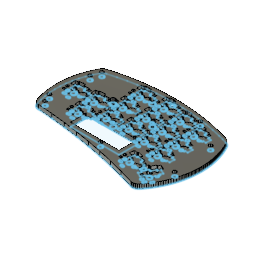
wubmeat-back (Autodesk Fusion 360 design; units mm, degrees)
Autodesk Fusion 360 part; units mm, degrees
(part 1 of 7)
sketch "test (1)" plane through (0, 0, 0) normal (0, 0, 1) x (1, 0, 0)
  line L0 (83.4424, 85.5345) -> (83.3623, 80.9353)
  line L1 (97.0028, 84.2973) -> (92.5034, 84.3759)
  line L2 (96.886, 77.5985) -> (96.9026, 78.5483)
  spline S0 degree 3 poles (84.2605, 76.4435) (84.4967, 76.6798) (84.6294, 77.0003) (84.6294, 77.3344) knots 0 0 0 0 1 1 1 1
  spline S1 degree 3 poles (83.369, 76.0746) (83.7034, 76.0744) (84.024, 76.2072) (84.2605, 76.4435) knots 0 0 0 0 1 1 1 1
  spline S2 degree 3 poles (84.6294, 77.3344) (84.6294, 77.6686) (84.4967, 77.989) (84.2605, 78.2253) knots 0 0 0 0 1 1 1 1
  line L3 (99.1805, 61.506) -> (99.2606, 66.1052)
  spline S3 degree 3 poles (83.369, 78.5943) (83.7034, 78.5945) (84.024, 78.4617) (84.2605, 78.2253) knots 0 0 0 0 1 1 1 1
  line L4 (92.03, 85.8843) -> (91.5386, 86.3933)
  line L5 (91.5386, 86.3933) -> (86.5394, 86.4806)
  spline S4 degree 3 poles (84.2605, 78.2253) (84.4967, 77.989) (84.6294, 77.6686) (84.6294, 77.3344) knots 0 0 0 0 1 1 1 1
  line L6 (90.0901, 60.7148) -> (96.5894, 60.6011)
  spline S5 degree 3 poles (84.2605, 76.4435) (84.024, 76.2072) (83.7034, 76.0744) (83.369, 76.0746) knots 0 0 0 0 1 1 1 1
  spline S6 degree 3 poles (83.369, 76.0746) (83.0349, 76.0746) (82.7144, 76.2073) (82.4781, 76.4435) knots 0 0 0 0 1 1 1 1
  line L7 (86.002, 85.4895) -> (83.4424, 85.5345)
  spline S7 degree 3 poles (89.6162, 62.5901) (89.8898, 62.3539) (90.0648, 62.0236) (90.1066, 61.6646) knots 0 0 0 0 1 1 1 1
  line L8 (83.3623, 80.9353) -> (86.3916, 80.882)
  line L9 (90.4038, 78.662) -> (90.3867, 77.7122)
  spline S8 degree 3 poles (82.4781, 76.4435) (82.7144, 76.2073) (83.0349, 76.0746) (83.369, 76.0746) knots 0 0 0 0 1 1 1 1
  spline S9 degree 3 poles (84.6294, 77.3344) (84.6294, 77.0003) (84.4967, 76.6798) (84.2605, 76.4435) knots 0 0 0 0 1 1 1 1
  line L10 (83.369, 78.5943) -> (83.369, 78.5943)
  spline S10 degree 3 poles (91.8543, 67.5299) (91.762, 67.6256) (91.712, 67.7545) (91.7158, 67.8875) knots 0 0 0 0 1 1 1 1
  line L11 (96.6861, 66.1501) -> (96.7062, 67.2999)
  spline S11 degree 3 poles (89.8984, 79.0222) (89.7425, 79.1123) (89.5756, 79.1816) (89.4017, 79.2284) knots 0 0 0 0 1 1 1 1
  line L12 (91.2419, 69.3959) -> (86.2428, 69.4832)
  spline S12 degree 3 poles (88.9258, 79.9379) (89.2871, 79.9488) (89.6393, 79.8238) (89.9128, 79.5875) knots 0 0 0 0 1 1 1 1
  line L13 (96.606, 61.5509) -> (99.1805, 61.506)
  line L14 (91.7334, 68.8869) -> (91.2419, 69.3959)
  line L15 (86.0102, 85.9696) -> (86.002, 85.4895)
  spline S13 degree 3 poles (89.9128, 79.5875) (90.1866, 79.3514) (90.3618, 79.0211) (90.4038, 78.662) knots 0 0 0 0 1 1 1 1
  line L16 (99.2606, 66.1052) -> (96.6861, 66.1501)
  line L17 (99.4771, 78.5034) -> (99.5572, 83.1026)
  spline S14 degree 3 poles (83.369, 78.5943) (83.0349, 78.5943) (82.7144, 78.4616) (82.4781, 78.2253) knots 0 0 0 0 1 1 1 1
  spline S15 degree 3 poles (92.1509, 84.5273) (92.0586, 84.623) (92.0087, 84.7519) (92.0124, 84.8849) knots 0 0 0 0 1 1 1 1
  line L18 (86.5394, 86.4807) -> (86.0102, 85.9696)
  spline S16 degree 3 poles (82.4781, 78.2253) (82.2419, 77.989) (82.1092, 77.6686) (82.1092, 77.3344) knots 0 0 0 0 1 1 1 1
  line L19 (83.369, 78.5943) -> (83.369, 78.5943)
  spline S17 degree 3 poles (82.1092, 77.3344) (82.1092, 77.6686) (82.2419, 77.989) (82.4781, 78.2253) knots 0 0 0 0 1 1 1 1
  spline S18 degree 3 poles (82.4781, 78.2253) (82.7144, 78.4616) (83.0349, 78.5943) (83.369, 78.5943) knots 0 0 0 0 1 1 1 1
  line L20 (96.9827, 83.1475) -> (97.0028, 84.2973)
  spline S19 degree 3 poles (90.4027, 78.5943) (90.3779, 78.6287) (90.3521, 78.6623) (90.3252, 78.6951) knots 0 0 0 0 1 1 1 1
  spline S20 degree 3 poles (84.2605, 78.2253) (84.024, 78.4617) (83.7034, 78.5945) (83.369, 78.5943) knots 0 0 0 0 1 1 1 1
  spline S21 degree 3 poles (90.3252, 78.6951) (90.1978, 78.8223) (90.0543, 78.9323) (89.8984, 79.0222) knots 0 0 0 0 1 1 1 1
  line L21 (90.1066, 61.6646) -> (90.0901, 60.7148)
  spline S22 degree 3 poles (87.4117, 78.6951) (87.0254, 78.3087) (86.8085, 77.7847) (86.8086, 77.2383) knots 0 0 0 0 1 1 1 1
  line L22 (99.5572, 83.1026) -> (96.9827, 83.1475)
  spline S23 degree 3 poles (88.8684, 79.2987) (88.322, 79.2986) (87.798, 79.0815) (87.4117, 78.6951) knots 0 0 0 0 1 1 1 1
  spline S24 degree 3 poles (89.4017, 79.2284) (89.2278, 79.275) (89.0485, 79.2986) (88.8684, 79.2987) knots 0 0 0 0 1 1 1 1
  spline S25 degree 3 poles (86.8086, 77.2383) (86.8085, 76.692) (87.0254, 76.168) (87.4117, 75.7816) knots 0 0 0 0 1 1 1 1
  spline S26 degree 3 poles (82.4781, 76.4435) (82.2419, 76.6798) (82.1092, 77.0003) (82.1092, 77.3344) knots 0 0 0 0 1 1 1 1
  spline S27 degree 3 poles (92.5034, 84.3759) (92.3703, 84.3769) (92.2433, 84.4315) (92.1509, 84.5273) knots 0 0 0 0 1 1 1 1
  spline S28 degree 3 poles (92.2067, 67.3785) (92.0737, 67.3795) (91.9467, 67.4341) (91.8543, 67.5299) knots 0 0 0 0 1 1 1 1
  spline S29 degree 3 poles (87.4117, 75.7816) (87.7981, 75.3953) (88.3221, 75.1784) (88.8684, 75.1785) knots 0 0 0 0 1 1 1 1
  line L23 (96.9026, 78.5483) -> (99.4771, 78.5034)
  line L24 (92.0124, 84.8849) -> (92.03, 85.8843)
  spline S30 degree 3 poles (82.1092, 77.3344) (82.1092, 77.0003) (82.2419, 76.6798) (82.4781, 76.4435) knots 0 0 0 0 1 1 1 1
  line L25 (90.3867, 77.7122) -> (96.886, 77.5985)
  line L26 (96.5894, 60.6011) -> (96.606, 61.5509)
  line L27 (87.3259, 79.9658) -> (88.9258, 79.9379)
  line L28 (86.3916, 80.882) -> (87.3259, 79.9658)
  line L29 (91.7158, 67.8875) -> (91.7334, 68.8869)
  spline S31 degree 3 poles (90.3252, 75.7816) (90.4524, 75.9089) (90.5624, 76.0524) (90.6523, 76.2084) knots 0 0 0 0 1 1 1 1
  line L30 (33.6537, 35.5701) -> (33.5768, 36.4532)
  spline S32 degree 3 poles (27.1038, 35.6595) (26.9779, 35.7005) (26.8465, 35.7214) (26.7141, 35.7215) knots 0 0 0 0 1 1 1 1
  line L31 (90.8673, 77.7039) -> (90.3867, 77.7122)
  spline S33 degree 3 poles (70.73, 73.4437) (71.0515, 73.4438) (71.3486, 73.6154) (71.5093, 73.8938) knots 0 0 0 0 1 1 1 1
  spline S34 degree 3 poles (87.3254, 70.9152) (87.1701, 71.1959) (87.176, 71.5381) (87.3409, 71.8133) knots 0 0 0 0 1 1 1 1
  line L32 (89.4048, 70.4279) -> (88.0949, 70.4511)
  spline S35 degree 3 poles (34.1829, 34.4074) (34.2296, 34.5813) (34.2532, 34.7606) (34.2532, 34.9407) knots 0 0 0 0 1 1 1 1
  spline S36 degree 3 poles (34.1829, 35.474) (34.1656, 35.5204) (34.1467, 35.5663) (34.1261, 35.6114) knots 0 0 0 0 1 1 1 1
  spline S37 degree 3 poles (90.1898, 70.8651) (90.0248, 70.5898) (89.7257, 70.4232) (89.4048, 70.4279) knots 0 0 0 0 1 1 1 1
  line L33 (72.5852, 72.4438) -> (73.0849, 71.9436)
  spline S38 degree 3 poles (27.9125, 34.8507) (27.8717, 34.9764) (27.8113, 35.0948) (27.7337, 35.2016) knots 0 0 0 0 1 1 1 1
  spline S39 degree 3 poles (88.8684, 75.1785) (89.0485, 75.1785) (89.2278, 75.2021) (89.4017, 75.2488) knots 0 0 0 0 1 1 1 1
  spline S40 degree 3 poles (27.7337, 33.7206) (27.8114, 33.8276) (27.8717, 33.9462) (27.9125, 34.072) knots 0 0 0 0 1 1 1 1
  spline S41 degree 3 poles (27.974, 34.4611) (27.9741, 34.5934) (27.9533, 34.7249) (27.9125, 34.8507) knots 0 0 0 0 1 1 1 1
  line L34 (69.42, 73.4437) -> (70.73, 73.4437)
  spline S42 degree 3 poles (68.6407, 73.8938) (68.8015, 73.6154) (69.0985, 73.4438) (69.42, 73.4437) knots 0 0 0 0 1 1 1 1
  spline S43 degree 3 poles (33.9772, 33.9107) (34.0672, 34.0666) (34.1363, 34.2335) (34.1829, 34.4074) knots 0 0 0 0 1 1 1 1
  line L35 (34.1261, 35.6114) -> (33.6537, 35.5701)
  spline S44 degree 3 poles (68.6407, 74.7935) (68.4801, 74.5151) (68.4801, 74.1722) (68.6407, 73.8938) knots 0 0 0 0 1 1 1 1
  spline S45 degree 3 poles (87.3409, 71.8133) (87.506, 72.0887) (87.8053, 72.2553) (88.1264, 72.2505) knots 0 0 0 0 1 1 1 1
  spline S46 degree 3 poles (93.3219, 77.661) (93.2123, 77.5064) (93.139, 77.3291) (93.1075, 77.1422) knots 0 0 0 0 1 1 1 1
  line L36 (67.585, 72.4438) -> (72.5852, 72.4438)
  spline S47 degree 3 poles (26.7141, 35.7215) (26.3799, 35.7214) (26.0594, 35.5884) (25.8232, 35.352) knots 0 0 0 0 1 1 1 1
  line L37 (26.7141, 35.7215) -> (26.7141, 35.7215)
  line L38 (73.0849, 71.9436) -> (73.0849, 70.9436)
  spline S48 degree 3 poles (89.4017, 75.2488) (89.5756, 75.2954) (89.7425, 75.3645) (89.8984, 75.4545) knots 0 0 0 0 1 1 1 1
  spline S49 degree 3 poles (90.8585, 76.705) (90.905, 76.879) (90.9284, 77.0583) (90.9283, 77.2383) knots 0 0 0 0 1 1 1 1
  spline S50 degree 3 poles (25.8232, 33.5702) (26.0595, 33.3339) (26.38, 33.2012) (26.7141, 33.2012) knots 0 0 0 0 1 1 1 1
  spline S51 degree 3 poles (33.2233, 33.1568) (33.3791, 33.2467) (33.5224, 33.3567) (33.6496, 33.4839) knots 0 0 0 0 1 1 1 1
  spline S52 degree 3 poles (88.0949, 70.4511) (87.774, 70.4576) (87.4808, 70.6344) (87.3254, 70.9152) knots 0 0 0 0 1 1 1 1
  spline S53 degree 3 poles (25.4543, 34.4611) (25.4542, 34.127) (25.587, 33.8065) (25.8232, 33.5702) knots 0 0 0 0 1 1 1 1
  spline S54 degree 3 poles (89.8984, 75.4545) (90.0543, 75.5444) (90.1978, 75.6543) (90.3252, 75.7816) knots 0 0 0 0 1 1 1 1
  spline S55 degree 3 poles (26.7141, 33.2012) (26.8464, 33.2011) (26.9779, 33.2219) (27.1038, 33.2627) knots 0 0 0 0 1 1 1 1
  spline S56 degree 3 poles (27.9125, 34.072) (27.9533, 34.1977) (27.974, 34.329) (27.974, 34.4611) knots 0 0 0 0 1 1 1 1
  spline S57 degree 3 poles (27.4546, 35.4807) (27.3478, 35.5583) (27.2294, 35.6186) (27.1038, 35.6595) knots 0 0 0 0 1 1 1 1
  spline S58 degree 3 poles (93.4764, 76.2513) (93.7129, 76.0149) (94.0335, 75.8822) (94.3679, 75.8823) knots 0 0 0 0 1 1 1 1
  spline S59 degree 3 poles (90.9283, 77.2383) (90.9258, 77.3953) (90.9053, 77.5516) (90.8673, 77.7039) knots 0 0 0 0 1 1 1 1
  spline S60 degree 3 poles (34.2532, 34.9407) (34.2532, 35.1207) (34.2296, 35.3) (34.1829, 35.474) knots 0 0 0 0 1 1 1 1
  spline S61 degree 3 poles (25.8232, 35.352) (25.587, 35.1157) (25.4542, 34.7952) (25.4543, 34.4611) knots 0 0 0 0 1 1 1 1
  spline S62 degree 3 poles (33.6496, 33.4839) (33.777, 33.6112) (33.8872, 33.7548) (33.9772, 33.9107) knots 0 0 0 0 1 1 1 1
  spline S63 degree 3 poles (69.42, 75.2436) (69.0985, 75.2435) (68.8015, 75.072) (68.6407, 74.7935) knots 0 0 0 0 1 1 1 1
  spline S64 degree 3 poles (93.1075, 77.1422) (93.1075, 76.8081) (93.2402, 76.4876) (93.4764, 76.2513) knots 0 0 0 0 1 1 1 1
  spline S65 degree 3 poles (90.6523, 76.2084) (90.7425, 76.3642) (90.8118, 76.5312) (90.8585, 76.705) knots 0 0 0 0 1 1 1 1
  spline S66 degree 3 poles (27.1038, 33.2627) (27.2294, 33.3037) (27.3478, 33.3642) (27.4546, 33.442) knots 0 0 0 0 1 1 1 1
  spline S67 degree 3 poles (90.2058, 71.7637) (90.3612, 71.4828) (90.3551, 71.1403) (90.1898, 70.8651) knots 0 0 0 0 1 1 1 1
  line L39 (90.3867, 77.7122) -> (90.4027, 78.5943)
  spline S68 degree 3 poles (89.4359, 72.2278) (89.7569, 72.2215) (90.0503, 72.0447) (90.2058, 71.7637) knots 0 0 0 0 1 1 1 1
  spline S69 degree 3 poles (27.7337, 35.2016) (27.6559, 35.3087) (27.5617, 35.4029) (27.4546, 35.4807) knots 0 0 0 0 1 1 1 1
  spline S70 degree 3 poles (27.4546, 33.442) (27.5617, 33.5197) (27.6559, 33.6137) (27.7337, 33.7206) knots 0 0 0 0 1 1 1 1
  line L40 (78.0851, 70.4434) -> (78.0851, 69.2936)
  line L41 (64.5051, 66.8436) -> (64.5051, 71.4438)
  line L42 (49.491, 73.2034) -> (49.491, 73.2034)
  spline S71 degree 3 poles (49.491, 73.2034) (49.8122, 73.2203) (50.1179, 73.0644) (50.293, 72.7947) knots 0 0 0 0 1 1 1 1
  spline S72 degree 3 poles (50.3401, 71.896) (50.1941, 71.6094) (49.9063, 71.4224) (49.5851, 71.4056) knots 0 0 0 0 1 1 1 1
  line L43 (49.5851, 71.4056) -> (48.2771, 71.3374)
  spline S73 degree 3 poles (102.8154, 73.1207) (102.9225, 73.0431) (103.0166, 72.9491) (103.0944, 72.8422) knots 0 0 0 0 1 1 1 1
  spline S74 degree 3 poles (103.2733, 72.4908) (103.314, 72.3651) (103.3348, 72.2338) (103.3347, 72.1017) knots 0 0 0 0 1 1 1 1
  spline S75 degree 3 poles (102.9658, 71.2103) (102.7295, 70.974) (102.409, 70.8413) (102.0749, 70.8413) knots 0 0 0 0 1 1 1 1
  spline S76 degree 3 poles (50.293, 72.7947) (50.4681, 72.525) (50.486, 72.1825) (50.3401, 71.896) knots 0 0 0 0 1 1 1 1
  line L44 (67.0651, 71.4438) -> (67.0651, 71.9234)
  spline S77 degree 3 poles (49.5851, 71.4056) (49.9063, 71.4224) (50.1941, 71.6094) (50.3401, 71.896) knots 0 0 0 0 1 1 1 1
  spline S78 degree 3 poles (100.815, 72.1017) (100.815, 72.4358) (100.9477, 72.7563) (101.184, 72.9926) knots 0 0 0 0 1 1 1 1
  line L45 (73.5851, 70.4434) -> (78.0851, 70.4434)
  spline S79 degree 3 poles (71.0783, 65.6106) (70.8006, 65.842) (70.4462, 65.9607) (70.0851, 65.9434) knots 0 0 0 0 1 1 1 1
  line L46 (68.4852, 65.9434) -> (67.5349, 66.8436)
  spline S80 degree 3 poles (48.1826, 73.1347) (47.8615, 73.1177) (47.574, 72.9308) (47.4281, 72.6443) knots 0 0 0 0 1 1 1 1
  line L47 (48.2771, 71.3374) -> (49.5851, 71.4056)
  line L48 (48.1826, 73.1347) -> (49.491, 73.2034)
  spline S81 degree 3 poles (102.4645, 73.2995) (102.5901, 73.2587) (102.7085, 73.1984) (102.8154, 73.1207) knots 0 0 0 0 1 1 1 1
  spline S82 degree 3 poles (103.3347, 72.1017) (103.3349, 71.7674) (103.2022, 71.4467) (102.9658, 71.2103) knots 0 0 0 0 1 1 1 1
  spline S83 degree 3 poles (71.5853, 64.6934) (71.5371, 65.0518) (71.3562, 65.3792) (71.0783, 65.6106) knots 0 0 0 0 1 1 1 1
  line L49 (78.0851, 64.6934) -> (78.0851, 63.7435)
  spline S84 degree 3 poles (101.184, 71.2103) (100.9476, 71.4467) (100.8149, 71.7674) (100.815, 72.1017) knots 0 0 0 0 1 1 1 1
  spline S85 degree 3 poles (73.2301, 70.5886) (73.3241, 70.4944) (73.4521, 70.4421) (73.5851, 70.4434) knots 0 0 0 0 1 1 1 1
  line L50 (49.491, 73.2034) -> (48.1826, 73.1347)
  spline S86 degree 3 poles (102.0749, 73.3616) (102.2072, 73.3615) (102.3387, 73.3405) (102.4645, 73.2995) knots 0 0 0 0 1 1 1 1
  spline S87 degree 3 poles (102.0749, 70.8413) (101.7407, 70.8413) (101.4203, 70.974) (101.184, 71.2103) knots 0 0 0 0 1 1 1 1
  line L51 (78.0851, 63.7435) -> (71.5853, 63.7435)
  line L52 (71.5853, 63.7435) -> (71.5853, 64.6934)
  line L53 (80.6602, 69.2936) -> (80.6602, 64.6934)
  line L54 (64.5051, 71.4438) -> (67.0651, 71.4438)
  line L55 (67.0651, 71.9234) -> (67.585, 72.4438)
  line L56 (67.5349, 66.8436) -> (64.5051, 66.8436)
  spline S88 degree 3 poles (47.4751, 71.7456) (47.6504, 71.4761) (47.9561, 71.3204) (48.2771, 71.3374) knots 0 0 0 0 1 1 1 1
  spline S89 degree 3 poles (47.4751, 71.7456) (47.3001, 72.0153) (47.2821, 72.3578) (47.4281, 72.6443) knots 0 0 0 0 1 1 1 1
  spline S90 degree 3 poles (103.0944, 72.8422) (103.1721, 72.7352) (103.2325, 72.6166) (103.2733, 72.4908) knots 0 0 0 0 1 1 1 1
  spline S91 degree 3 poles (50.3401, 71.896) (50.486, 72.1825) (50.4681, 72.525) (50.293, 72.7947) knots 0 0 0 0 1 1 1 1
  line L57 (80.6602, 64.6934) -> (78.0851, 64.6934)
  line L58 (70.0851, 65.9434) -> (68.4852, 65.9434)
  line L59 (88.1264, 72.2505) -> (88.1264, 72.2505)
  spline S92 degree 3 poles (73.0849, 70.9436) (73.0836, 70.8106) (73.136, 70.6826) (73.2301, 70.5886) knots 0 0 0 0 1 1 1 1
  line L60 (78.0851, 69.2936) -> (80.6602, 69.2936)
  spline S93 degree 3 poles (48.2771, 71.3374) (47.9561, 71.3204) (47.6504, 71.4761) (47.4751, 71.7456) knots 0 0 0 0 1 1 1 1
  spline S94 degree 3 poles (47.4281, 72.6443) (47.574, 72.9308) (47.8615, 73.1177) (48.1826, 73.1347) knots 0 0 0 0 1 1 1 1
  spline S95 degree 3 poles (50.293, 72.7947) (50.1179, 73.0644) (49.8122, 73.2203) (49.491, 73.2034) knots 0 0 0 0 1 1 1 1
  spline S96 degree 3 poles (47.4281, 72.6443) (47.2821, 72.3578) (47.3001, 72.0153) (47.4751, 71.7456) knots 0 0 0 0 1 1 1 1
  spline S97 degree 3 poles (110.1416, 22.527) (109.6775, 22.5269) (109.2325, 22.3425) (108.9044, 22.0143) knots 0 0 0 0 1 1 1 1
  spline S98 degree 3 poles (108.9044, 19.5395) (109.2325, 19.2114) (109.6775, 19.027) (110.1416, 19.0269) knots 0 0 0 0 1 1 1 1
  spline S99 degree 3 poles (108.9044, 22.0143) (108.5762, 21.6861) (108.3918, 21.2409) (108.3918, 20.7767) knots 0 0 0 0 1 1 1 1
  spline S100 degree 3 poles (111.3792, 19.5395) (111.7074, 19.8676) (111.8917, 20.3126) (111.8918, 20.7767) knots 0 0 0 0 1 1 1 1
  line L61 (102.0749, 73.3616) -> (102.0749, 73.3616)
  spline S101 degree 3 poles (111.8918, 20.7767) (111.8918, 20.9297) (111.8716, 21.0821) (111.8319, 21.2299) knots 0 0 0 0 1 1 1 1
  spline S102 degree 3 poles (111.017, 22.2923) (110.8845, 22.3688) (110.7425, 22.4275) (110.5948, 22.467) knots 0 0 0 0 1 1 1 1
  spline S103 degree 3 poles (110.5948, 22.467) (110.447, 22.5067) (110.2946, 22.5269) (110.1416, 22.527) knots 0 0 0 0 1 1 1 1
  spline S104 degree 3 poles (111.6572, 21.6516) (111.5808, 21.7841) (111.4873, 21.9061) (111.3792, 22.0143) knots 0 0 0 0 1 1 1 1
  line L62 (110.1416, 22.527) -> (110.1416, 22.527)
  spline S105 degree 3 poles (102.6366, 18.7768) (102.4002, 18.5406) (102.2672, 18.2201) (102.2671, 17.8859) knots 0 0 0 0 1 1 1 1
  spline S106 degree 3 poles (103.5275, 19.1458) (103.1934, 19.1458) (102.8729, 19.013) (102.6366, 18.7768) knots 0 0 0 0 1 1 1 1
  spline S107 degree 3 poles (102.2671, 17.8859) (102.2672, 17.5517) (102.4002, 17.2312) (102.6366, 16.995) knots 0 0 0 0 1 1 1 1
  spline S108 degree 3 poles (108.3918, 20.7767) (108.3919, 20.3126) (108.5763, 19.8676) (108.9044, 19.5395) knots 0 0 0 0 1 1 1 1
  spline S109 degree 3 poles (111.3792, 22.0143) (111.2711, 22.1224) (111.1493, 22.2159) (111.017, 22.2923) knots 0 0 0 0 1 1 1 1
  spline S110 degree 3 poles (111.8319, 21.2299) (111.7923, 21.3775) (111.7336, 21.5192) (111.6572, 21.6516) knots 0 0 0 0 1 1 1 1
  spline S111 degree 3 poles (103.5275, 16.626) (103.8616, 16.626) (104.1821, 16.7587) (104.4184, 16.995) knots 0 0 0 0 1 1 1 1
  spline S112 degree 3 poles (110.1416, 19.0269) (110.6058, 19.0269) (111.051, 19.2113) (111.3792, 19.5395) knots 0 0 0 0 1 1 1 1
  spline S113 degree 3 poles (102.6366, 16.995) (102.8729, 16.7587) (103.1934, 16.626) (103.5275, 16.626) knots 0 0 0 0 1 1 1 1
  spline S114 degree 3 poles (104.7874, 17.8859) (104.7874, 18.018) (104.7666, 18.1493) (104.7259, 18.275) knots 0 0 0 0 1 1 1 1
  spline S115 degree 3 poles (101.184, 72.9926) (101.4203, 73.2288) (101.7407, 73.3616) (102.0749, 73.3616) knots 0 0 0 0 1 1 1 1
  line L63 (88.1264, 72.2505) -> (89.4359, 72.2278)
  spline S116 degree 3 poles (118.1344, 12.6071) (118.0087, 12.6481) (117.8774, 12.669) (117.7452, 12.6692) knots 0 0 0 0 1 1 1 1
  line L64 (117.7452, 12.6692) -> (117.7452, 12.6692)
  spline S117 degree 3 poles (117.7452, 12.6692) (117.8774, 12.669) (118.0087, 12.6481) (118.1344, 12.6071) knots 0 0 0 0 1 1 1 1
  spline S118 degree 3 poles (103.9166, 19.0843) (103.7909, 19.125) (103.6596, 19.1458) (103.5275, 19.1458) knots 0 0 0 0 1 1 1 1
  spline S119 degree 3 poles (96.6716, 20.3922) (96.2853, 20.0058) (96.0684, 19.4818) (96.0685, 18.9354) knots 0 0 0 0 1 1 1 1
  line L65 (44.388, 75.0385) -> (43.0795, 74.9702)
  spline S120 degree 3 poles (119.0051, 11.4088) (119.0051, 11.0746) (118.8724, 10.7542) (118.6361, 10.5179) knots 0 0 0 0 1 1 1 1
  line L66 (131.3718, 31.3068) -> (131.3718, 31.3068)
  spline S121 degree 3 poles (104.5466, 18.6264) (104.4689, 18.7335) (104.3749, 18.8276) (104.268, 18.9055) knots 0 0 0 0 1 1 1 1
  spline S122 degree 3 poles (42.3721, 73.5812) (42.5472, 73.3114) (42.8529, 73.1556) (43.1741, 73.1724) knots 0 0 0 0 1 1 1 1
  spline S123 degree 3 poles (104.4184, 16.995) (104.6547, 17.2313) (104.7874, 17.5517) (104.7874, 17.8859) knots 0 0 0 0 1 1 1 1
  spline S124 degree 3 poles (116.4848, 11.4088) (116.485, 11.743) (116.6179, 12.0635) (116.8543, 12.2997) knots 0 0 0 0 1 1 1 1
  spline S125 degree 3 poles (132.6089, 30.7941) (132.5008, 30.9022) (132.379, 30.9957) (132.2467, 31.0722) knots 0 0 0 0 1 1 1 1
  spline S126 degree 3 poles (118.4858, 12.4283) (118.5927, 12.3505) (118.6867, 12.2564) (118.7643, 12.1493) knots 0 0 0 0 1 1 1 1
  spline S127 degree 3 poles (116.8543, 10.5179) (116.6179, 10.7541) (116.485, 11.0746) (116.4848, 11.4088) knots 0 0 0 0 1 1 1 1
  spline S128 degree 3 poles (116.8543, 12.2997) (117.0905, 12.5361) (117.411, 12.669) (117.7452, 12.6692) knots 0 0 0 0 1 1 1 1
  spline S129 degree 3 poles (96.0685, 18.9354) (96.0684, 18.3891) (96.2853, 17.8651) (96.6716, 17.4787) knots 0 0 0 0 1 1 1 1
  spline S130 degree 3 poles (44.482, 73.2412) (44.8032, 73.258) (45.0911, 73.4449) (45.237, 73.7316) knots 0 0 0 0 1 1 1 1
  spline S131 degree 3 poles (125.6832, 15.2519) (125.3626, 15.2296) (125.0781, 15.038) (124.937, 14.7491) knots 0 0 0 0 1 1 1 1
  spline S132 degree 3 poles (43.9735, 78.7654) (43.7372, 79.0016) (43.4168, 79.1343) (43.0826, 79.1343) knots 0 0 0 0 1 1 1 1
  line L67 (103.5275, 19.1458) -> (103.5275, 19.1458)
  spline S133 degree 3 poles (43.0795, 74.9702) (42.7585, 74.9533) (42.4709, 74.7663) (42.3251, 74.4798) knots 0 0 0 0 1 1 1 1
  spline S134 degree 3 poles (132.2467, 31.0722) (132.1142, 31.1488) (131.9723, 31.2077) (131.8245, 31.2473) knots 0 0 0 0 1 1 1 1
  line L68 (124.937, 14.7491) -> (124.3629, 13.5719)
  spline S135 degree 3 poles (124.3629, 13.5719) (124.223, 13.283) (124.2476, 12.9413) (124.4275, 12.6754) knots 0 0 0 0 1 1 1 1
  line L69 (117.7452, 12.6692) -> (117.7452, 12.6692)
  spline S136 degree 3 poles (130.1341, 28.3194) (130.4624, 27.9911) (130.9076, 27.8067) (131.3718, 27.8067) knots 0 0 0 0 1 1 1 1
  spline S137 degree 3 poles (124.4275, 12.6754) (124.6072, 12.4096) (124.9147, 12.2596) (125.2347, 12.2816) knots 0 0 0 0 1 1 1 1
  line L70 (125.9809, 12.7828) -> (126.555, 13.96)
  line L71 (44.388, 75.0385) -> (44.388, 75.0385)
  spline S138 degree 3 poles (96.6716, 17.4787) (97.0579, 17.0922) (97.5819, 16.8751) (98.1283, 16.8751) knots 0 0 0 0 1 1 1 1
  spline S139 degree 3 poles (99.1583, 17.1516) (99.3142, 17.2415) (99.4577, 17.3515) (99.5851, 17.4787) knots 0 0 0 0 1 1 1 1
  spline S140 degree 3 poles (42.3251, 74.4798) (42.1791, 74.1934) (42.197, 73.8508) (42.3721, 73.5812) knots 0 0 0 0 1 1 1 1
  line L72 (43.1741, 73.1724) -> (44.482, 73.2412)
  spline S141 degree 3 poles (104.268, 18.9055) (104.161, 18.9831) (104.0424, 19.0435) (103.9166, 19.0843) knots 0 0 0 0 1 1 1 1
  spline S142 degree 3 poles (99.9122, 17.9055) (100.0023, 18.0613) (100.0717, 18.2283) (100.1184, 18.4021) knots 0 0 0 0 1 1 1 1
  spline S143 degree 3 poles (45.237, 73.7316) (45.383, 74.018) (45.365, 74.3606) (45.19, 74.6302) knots 0 0 0 0 1 1 1 1
  spline S144 degree 3 poles (98.1283, 16.8751) (98.3084, 16.8751) (98.4877, 16.8987) (98.6616, 16.9454) knots 0 0 0 0 1 1 1 1
  spline S145 degree 3 poles (43.9735, 76.9836) (44.2098, 77.2199) (44.3425, 77.5403) (44.3425, 77.8745) knots 0 0 0 0 1 1 1 1
  spline S146 degree 3 poles (99.5851, 17.4787) (99.7123, 17.6061) (99.8223, 17.7496) (99.9122, 17.9055) knots 0 0 0 0 1 1 1 1
  spline S147 degree 3 poles (132.6089, 28.3194) (132.9372, 28.6476) (133.1216, 29.0928) (133.1215, 29.557) knots 0 0 0 0 1 1 1 1
  spline S148 degree 3 poles (133.1215, 29.557) (133.1216, 29.7099) (133.1016, 29.862) (133.0621, 30.0097) knots 0 0 0 0 1 1 1 1
  spline S149 degree 3 poles (130.1341, 30.7941) (129.806, 30.466) (129.6216, 30.021) (129.6215, 29.557) knots 0 0 0 0 1 1 1 1
  spline S150 degree 3 poles (133.0621, 30.0097) (133.0226, 30.1575) (132.9639, 30.2994) (132.8875, 30.4319) knots 0 0 0 0 1 1 1 1
  spline S151 degree 3 poles (131.3718, 31.3068) (130.9076, 31.3068) (130.4624, 31.1224) (130.1341, 30.7941) knots 0 0 0 0 1 1 1 1
  spline S152 degree 3 poles (131.3718, 27.8067) (131.8358, 27.8068) (132.2808, 27.9912) (132.6089, 28.3194) knots 0 0 0 0 1 1 1 1
  spline S153 degree 3 poles (100.1184, 18.4021) (100.1649, 18.5761) (100.1883, 18.7554) (100.1882, 18.9354) knots 0 0 0 0 1 1 1 1
  spline S154 degree 3 poles (131.8245, 31.2473) (131.6768, 31.2868) (131.5246, 31.3068) (131.3718, 31.3068) knots 0 0 0 0 1 1 1 1
  spline S155 degree 3 poles (118.9436, 11.7984) (118.9844, 11.6726) (119.0052, 11.5411) (119.0051, 11.4088) knots 0 0 0 0 1 1 1 1
  spline S156 degree 3 poles (100.1882, 18.9354) (100.1883, 19.1155) (100.1649, 19.2948) (100.1184, 19.4687) knots 0 0 0 0 1 1 1 1
  spline S157 degree 3 poles (45.19, 74.6302) (45.0148, 74.8998) (44.709, 75.0554) (44.388, 75.0385) knots 0 0 0 0 1 1 1 1
  spline S158 degree 3 poles (98.6616, 16.9454) (98.8355, 16.9921) (99.0024, 17.0614) (99.1583, 17.1516) knots 0 0 0 0 1 1 1 1
  line L73 (43.0826, 79.1343) -> (43.0826, 79.1343)
  spline S159 degree 3 poles (44.3425, 77.8745) (44.3425, 78.2086) (44.2098, 78.5291) (43.9735, 78.7654) knots 0 0 0 0 1 1 1 1
  spline S160 degree 3 poles (118.7643, 12.1493) (118.8421, 12.0425) (118.9026, 11.924) (118.9436, 11.7984) knots 0 0 0 0 1 1 1 1
  spline S161 degree 3 poles (100.1184, 19.4687) (100.0717, 19.6426) (100.0023, 19.8095) (99.9122, 19.9654) knots 0 0 0 0 1 1 1 1
  spline S162 degree 3 poles (132.8875, 30.4319) (132.8108, 30.5643) (132.7172, 30.6861) (132.6089, 30.7941) knots 0 0 0 0 1 1 1 1
  spline S163 degree 3 poles (118.1344, 12.6071) (118.2601, 12.5664) (118.3787, 12.506) (118.4858, 12.4283) knots 0 0 0 0 1 1 1 1
  spline S164 degree 3 poles (117.7452, 10.1489) (117.4111, 10.1489) (117.0906, 10.2816) (116.8543, 10.5179) knots 0 0 0 0 1 1 1 1
  spline S165 degree 3 poles (98.1283, 20.9953) (97.582, 20.9954) (97.058, 20.7784) (96.6716, 20.3922) knots 0 0 0 0 1 1 1 1
  spline S166 degree 3 poles (118.6361, 10.5179) (118.3998, 10.2816) (118.0794, 10.1489) (117.7452, 10.1489) knots 0 0 0 0 1 1 1 1
  spline S167 degree 3 poles (129.6215, 29.557) (129.6215, 29.0928) (129.8059, 28.6476) (130.1341, 28.3194) knots 0 0 0 0 1 1 1 1
  spline S168 degree 3 poles (104.7259, 18.275) (104.6849, 18.4008) (104.6244, 18.5194) (104.5466, 18.6264) knots 0 0 0 0 1 1 1 1
  spline S169 degree 3 poles (120.6892, 18.3422) (120.6522, 18.348) (120.6149, 18.3529) (120.5776, 18.3567) knots 0 0 0 0 1 1 1 1
  line L74 (120.3688, 17.9288) -> (119.7348, 18.2378)
  line L75 (102.5524, 25.9195) -> (102.743, 26.9014)
  spline S170 degree 3 poles (117.7452, 12.6692) (117.411, 12.669) (117.0905, 12.5361) (116.8543, 12.2997) knots 0 0 0 0 1 1 1 1
  spline S171 degree 3 poles (123.827, 21.2955) (123.8271, 21.4278) (123.8064, 21.5593) (123.7655, 21.6851) knots 0 0 0 0 1 1 1 1
  spline S172 degree 3 poles (118.6997, 14.8959) (119.0859, 14.5096) (119.6097, 14.2925) (120.1559, 14.2923) knots 0 0 0 0 1 1 1 1
  line L76 (126.555, 13.96) -> (125.9809, 12.7828)
  line L77 (120.5776, 18.3567) -> (120.3688, 17.9288)
  spline S173 degree 3 poles (118.6361, 10.5179) (118.8724, 10.7542) (119.0051, 11.0746) (119.0051, 11.4088) knots 0 0 0 0 1 1 1 1
  spline S174 degree 3 poles (118.9436, 11.7984) (118.9026, 11.924) (118.8421, 12.0425) (118.7643, 12.1493) knots 0 0 0 0 1 1 1 1
  spline S175 degree 3 poles (99.8487, 20.4961) (99.8826, 20.357) (99.8956, 20.2137) (99.8874, 20.0708) knots 0 0 0 0 1 1 1 1
  spline S176 degree 3 poles (121.6303, 20.5152) (121.6438, 20.4776) (121.6592, 20.4407) (121.6763, 20.4046) knots 0 0 0 0 1 1 1 1
  spline S177 degree 3 poles (119.0051, 11.4088) (119.0052, 11.5411) (118.9844, 11.6726) (118.9436, 11.7984) knots 0 0 0 0 1 1 1 1
  spline S178 degree 3 poles (125.2347, 12.2816) (125.555, 12.3036) (125.8394, 12.4946) (125.9809, 12.7828) knots 0 0 0 0 1 1 1 1
  spline S179 degree 3 poles (122.146, 16.8854) (122.0994, 17.0592) (122.0303, 17.2262) (121.9403, 17.382) knots 0 0 0 0 1 1 1 1
  spline S180 degree 3 poles (116.4848, 11.4088) (116.485, 11.0746) (116.6179, 10.7541) (116.8543, 10.5179) knots 0 0 0 0 1 1 1 1
  spline S181 degree 3 poles (116.8543, 12.2997) (116.6179, 12.0635) (116.485, 11.743) (116.4848, 11.4088) knots 0 0 0 0 1 1 1 1
  spline S182 degree 3 poles (118.4858, 12.4283) (118.3787, 12.506) (118.2601, 12.5664) (118.1344, 12.6071) knots 0 0 0 0 1 1 1 1
  line L78 (108.7954, 18.3391) -> (109.6734, 22.8546)
  spline S183 degree 3 poles (121.1858, 14.5683) (121.3418, 14.6583) (121.4853, 14.7685) (121.6127, 14.8959) knots 0 0 0 0 1 1 1 1
  line L79 (125.6832, 15.2519) -> (125.6832, 15.2519)
  spline S184 degree 3 poles (125.6832, 15.2519) (126.0039, 15.2744) (126.3122, 15.1241) (126.492, 14.8577) knots 0 0 0 0 1 1 1 1
  spline S185 degree 3 poles (99.6874, 20.8919) (99.7605, 20.7687) (99.8148, 20.6353) (99.8487, 20.4961) knots 0 0 0 0 1 1 1 1
  spline S186 degree 3 poles (126.492, 14.8577) (126.3122, 15.1241) (126.0039, 15.2744) (125.6832, 15.2519) knots 0 0 0 0 1 1 1 1
  spline S187 degree 3 poles (118.6997, 17.8089) (118.3133, 17.4226) (118.0961, 16.8986) (118.0961, 16.3521) knots 0 0 0 0 1 1 1 1
  spline S188 degree 3 poles (122.5672, 20.0356) (122.9013, 20.0356) (123.2218, 20.1683) (123.4581, 20.4046) knots 0 0 0 0 1 1 1 1
  spline S189 degree 3 poles (121.1858, 18.1365) (121.03, 18.2265) (120.863, 18.2956) (120.6892, 18.3422) knots 0 0 0 0 1 1 1 1
  spline S190 degree 3 poles (117.7452, 10.1489) (118.0794, 10.1489) (118.3998, 10.2816) (118.6361, 10.5179) knots 0 0 0 0 1 1 1 1
  spline S191 degree 3 poles (116.8543, 10.5179) (117.0906, 10.2816) (117.4111, 10.1489) (117.7452, 10.1489) knots 0 0 0 0 1 1 1 1
  line L80 (106.0865, 17.8978) -> (106.2679, 18.8305)
  spline S192 degree 3 poles (102.9477, 25.3335) (102.8169, 25.3575) (102.7012, 25.4331) (102.6268, 25.5433) knots 0 0 0 0 1 1 1 1
  spline S193 degree 3 poles (123.5867, 22.0365) (123.5089, 22.1435) (123.4147, 22.2375) (123.3077, 22.3151) knots 0 0 0 0 1 1 1 1
  spline S194 degree 3 poles (102.6268, 25.5433) (102.5524, 25.6536) (102.5256, 25.7892) (102.5524, 25.9195) knots 0 0 0 0 1 1 1 1
  spline S195 degree 3 poles (119.7348, 18.2378) (119.3567, 18.1932) (118.9985, 18.0448) (118.6997, 17.8089) knots 0 0 0 0 1 1 1 1
  spline S196 degree 3 poles (118.0961, 16.3521) (118.0963, 15.8059) (118.3134, 15.2821) (118.6997, 14.8959) knots 0 0 0 0 1 1 1 1
  line L81 (107.1454, 23.346) -> (107.365, 24.4746)
  line L82 (106.2679, 18.8305) -> (108.7954, 18.3391)
  spline S197 degree 3 poles (120.1559, 14.2923) (120.336, 14.2923) (120.5153, 14.316) (120.6892, 14.3626) knots 0 0 0 0 1 1 1 1
  spline S198 degree 3 poles (121.6127, 14.8959) (121.7401, 15.0231) (121.8502, 15.1664) (121.9403, 15.3222) knots 0 0 0 0 1 1 1 1
  spline S199 degree 3 poles (126.492, 14.8577) (126.6718, 14.5912) (126.6958, 14.249) (126.555, 13.96) knots 0 0 0 0 1 1 1 1
  line L83 (109.6734, 22.8546) -> (107.1454, 23.346)
  line L84 (102.743, 26.9014) -> (102.3477, 27.4874)
  line L85 (102.3477, 27.4874) -> (97.4395, 28.4413)
  spline S200 degree 3 poles (125.9809, 12.7828) (125.8394, 12.4946) (125.555, 12.3036) (125.2347, 12.2816) knots 0 0 0 0 1 1 1 1
  line L86 (99.706, 19.138) -> (106.0865, 17.8978)
  spline S201 degree 3 poles (123.3077, 22.3151) (123.2007, 22.3927) (123.0821, 22.4531) (122.9563, 22.4939) knots 0 0 0 0 1 1 1 1
  spline S202 degree 3 poles (120.6892, 14.3626) (120.863, 14.4092) (121.03, 14.4783) (121.1858, 14.5683) knots 0 0 0 0 1 1 1 1
  spline S203 degree 3 poles (122.146, 15.8194) (122.1926, 15.9931) (122.2162, 16.1722) (122.2163, 16.3521) knots 0 0 0 0 1 1 1 1
  spline S204 degree 3 poles (122.2163, 16.3521) (122.2163, 16.5322) (122.1926, 16.7115) (122.146, 16.8854) knots 0 0 0 0 1 1 1 1
  spline S205 degree 3 poles (121.6127, 17.8089) (121.4853, 17.9363) (121.3418, 18.0464) (121.1858, 18.1365) knots 0 0 0 0 1 1 1 1
  line L87 (122.6214, 22.5471) -> (121.6303, 20.5152)
  spline S206 degree 3 poles (121.9403, 15.3222) (122.0303, 15.4782) (122.0995, 15.6454) (122.146, 15.8194) knots 0 0 0 0 1 1 1 1
  spline S207 degree 3 poles (126.555, 13.96) (126.6958, 14.249) (126.6718, 14.5912) (126.492, 14.8577) knots 0 0 0 0 1 1 1 1
  spline S208 degree 3 poles (99.4177, 21.2232) (99.5235, 21.1267) (99.6144, 21.0151) (99.6874, 20.8919) knots 0 0 0 0 1 1 1 1
  spline S209 degree 3 poles (123.4581, 20.4046) (123.6943, 20.6409) (123.827, 20.9614) (123.827, 21.2955) knots 0 0 0 0 1 1 1 1
  spline S210 degree 3 poles (123.7655, 21.6851) (123.7247, 21.8109) (123.6644, 21.9295) (123.5867, 22.0365) knots 0 0 0 0 1 1 1 1
  spline S211 degree 3 poles (121.6763, 20.4046) (121.9126, 20.1683) (122.233, 20.0356) (122.5672, 20.0356) knots 0 0 0 0 1 1 1 1
  spline S212 degree 3 poles (122.9563, 22.4939) (122.8476, 22.5266) (122.7349, 22.5445) (122.6214, 22.5471) knots 0 0 0 0 1 1 1 1
  spline S213 degree 3 poles (121.9403, 17.382) (121.8502, 17.538) (121.7401, 17.6815) (121.6127, 17.8089) knots 0 0 0 0 1 1 1 1
  line L88 (107.365, 24.4746) -> (102.9477, 25.3335)
  line L89 (99.8874, 20.0708) -> (99.706, 19.138)
  spline S214 degree 3 poles (111.8815, 36.478) (112.2157, 36.4782) (112.5362, 36.6111) (112.7724, 36.8475) knots 0 0 0 0 1 1 1 1
  spline S215 degree 3 poles (107.842, 39.3869) (107.7146, 39.5141) (107.5711, 39.6241) (107.4151, 39.714) knots 0 0 0 0 1 1 1 1
  spline S216 degree 3 poles (106.918, 35.9406) (107.092, 35.9871) (107.2591, 36.0563) (107.4151, 36.1463) knots 0 0 0 0 1 1 1 1
  spline S217 degree 3 poles (106.3852, 35.8703) (106.5651, 35.8704) (106.7442, 35.894) (106.918, 35.9406) knots 0 0 0 0 1 1 1 1
  spline S218 degree 3 poles (102.5477, 88.5901) (99.8159, 89.0395) (97.0751, 89.4322) (94.327, 89.7678) knots 0 0 0 0 1 1 1 1
  spline S219 degree 3 poles (86.065, 90.6034) (83.3054, 90.8247) (80.5415, 90.9888) (77.7751, 91.0954) knots 0 0 0 0 1 1 1 1
  spline S220 degree 3 poles (91.3236, 7.5423) (95.8325, 6.4644) (100.3262, 5.3238) (104.8034, 4.1208) knots 0 0 0 0 1 1 1 1
  spline S221 degree 3 poles (120.9905, 0.1753) (121.4561, 0.2614) (121.9099, 0.4022) (122.3424, 0.595) knots 0 0 0 0 1 1 1 1
  spline S222 degree 3 poles (94.327, 89.7678) (91.5791, 90.1035) (88.8245, 90.3821) (86.065, 90.6034) knots 0 0 0 0 1 1 1 1
  spline S223 degree 3 poles (126.061, 4.2247) (126.3038, 4.5482) (126.5437, 4.8738) (126.7809, 5.2014) knots 0 0 0 0 1 1 1 1
  spline S224 degree 3 poles (127.4836, 6.1905) (127.7151, 6.5222) (127.9437, 6.8558) (128.1694, 7.1915) knots 0 0 0 0 1 1 1 1
  spline S225 degree 3 poles (126.7809, 5.2014) (127.018, 5.5291) (127.2522, 5.8588) (127.4836, 6.1905) knots 0 0 0 0 1 1 1 1
  spline S226 degree 3 poles (129.4882, 9.2285) (129.702, 9.5719) (129.9129, 9.9171) (130.1207, 10.2641) knots 0 0 0 0 1 1 1 1
  spline S227 degree 3 poles (110.6216, 37.7384) (110.6216, 37.4043) (110.7544, 37.0838) (110.9906, 36.8475) knots 0 0 0 0 1 1 1 1
  spline S228 degree 3 poles (118.7643, 12.1493) (118.6867, 12.2564) (118.5927, 12.3505) (118.4858, 12.4283) knots 0 0 0 0 1 1 1 1
  spline S229 degree 3 poles (131.3718, 27.8067) (130.9076, 27.8067) (130.4624, 27.9911) (130.1341, 28.3194) knots 0 0 0 0 1 1 1 1
  spline S230 degree 3 poles (104.7316, 31.6344) (104.8822, 31.3509) (105.1725, 31.1692) (105.4933, 31.1574) knots 0 0 0 0 1 1 1 1
  line L90 (106.8653, 32.9103) -> (105.5558, 32.9563)
  line L91 (131.3718, 31.3068) -> (131.3718, 31.3068)
  spline S231 degree 3 poles (77.7544, 10.5871) (82.2914, 9.6351) (86.8149, 8.6201) (91.3236, 7.5423) knots 0 0 0 0 1 1 1 1
  spline S232 degree 3 poles (107.6285, 32.4333) (107.4776, 32.7172) (107.1866, 32.8991) (106.8653, 32.9103) knots 0 0 0 0 1 1 1 1
  spline S233 degree 3 poles (128.1694, 7.1915) (128.395, 7.5271) (128.6178, 7.8648) (128.8376, 8.2043) knots 0 0 0 0 1 1 1 1
  spline S234 degree 3 poles (132.4689, 14.5104) (132.6522, 14.8709) (132.8324, 15.233) (133.0094, 15.5966) knots 0 0 0 0 1 1 1 1
  spline S235 degree 3 poles (107.9422, 39.2562) (107.9106, 39.3011) (107.8771, 39.3447) (107.842, 39.3869) knots 0 0 0 0 1 1 1 1
  spline S236 degree 3 poles (124.5712, 2.3096) (124.8249, 2.6245) (125.0759, 2.9417) (125.3241, 3.2609) knots 0 0 0 0 1 1 1 1
  spline S237 degree 3 poles (131.3315, 12.3668) (131.5273, 12.7207) (131.7201, 13.0763) (131.9097, 13.4335) knots 0 0 0 0 1 1 1 1
  spline S238 degree 3 poles (130.7351, 11.3101) (130.937, 11.6606) (131.1358, 12.0129) (131.3315, 12.3668) knots 0 0 0 0 1 1 1 1
  spline S239 degree 3 poles (64.1056, 13.2536) (68.6674, 12.4281) (73.2174, 11.5392) (77.7544, 10.5871) knots 0 0 0 0 1 1 1 1
  spline S240 degree 3 poles (128.8376, 8.2043) (129.0574, 8.5438) (129.2743, 8.8853) (129.4882, 9.2285) knots 0 0 0 0 1 1 1 1
  spline S241 degree 3 poles (130.1207, 10.2641) (130.3285, 10.611) (130.5333, 10.9597) (130.7351, 11.3101) knots 0 0 0 0 1 1 1 1
  spline S242 degree 3 poles (130.1341, 28.3194) (129.8059, 28.6476) (129.6215, 29.0928) (129.6215, 29.557) knots 0 0 0 0 1 1 1 1
  spline S243 degree 3 poles (131.9097, 13.4335) (132.0992, 13.7908) (132.2856, 14.1498) (132.4689, 14.5104) knots 0 0 0 0 1 1 1 1
  spline S244 degree 3 poles (134.0342, 17.7965) (134.1984, 18.166) (134.3595, 18.5368) (134.5173, 18.9091) knots 0 0 0 0 1 1 1 1
  spline S245 degree 3 poles (133.5313, 16.6922) (133.7021, 17.0588) (133.8697, 17.4269) (134.0342, 17.7965) knots 0 0 0 0 1 1 1 1
  spline S246 degree 3 poles (113.0799, 38.1275) (113.0687, 38.1513) (113.0568, 38.1748) (113.0442, 38.1978) knots 0 0 0 0 1 1 1 1
  spline S247 degree 3 poles (133.0094, 15.5966) (133.1866, 15.9603) (133.3605, 16.3255) (133.5313, 16.6922) knots 0 0 0 0 1 1 1 1
  spline S248 degree 3 poles (113.1419, 37.7384) (113.1418, 37.8706) (113.1208, 38.0019) (113.0799, 38.1275) knots 0 0 0 0 1 1 1 1
  line L92 (113.0442, 38.1978) -> (110.8438, 38.2748)
  spline S249 degree 3 poles (133.1215, 29.557) (133.1216, 29.0928) (132.9372, 28.6476) (132.6089, 28.3194) knots 0 0 0 0 1 1 1 1
  spline S250 degree 3 poles (123.5583, 1.32) (123.9338, 1.6087) (124.2738, 1.9409) (124.5712, 2.3096) knots 0 0 0 0 1 1 1 1
  spline S251 degree 3 poles (122.3424, 0.595) (122.7749, 0.7878) (123.183, 1.0312) (123.5583, 1.32) knots 0 0 0 0 1 1 1 1
  spline S252 degree 3 poles (106.918, 39.9202) (106.7442, 39.9668) (106.5651, 39.9904) (106.3852, 39.9905) knots 0 0 0 0 1 1 1 1
  spline S253 degree 3 poles (104.3249, 37.9301) (104.3249, 37.3837) (104.542, 36.8597) (104.9284, 36.4734) knots 0 0 0 0 1 1 1 1
  spline S254 degree 3 poles (104.8034, 4.1208) (109.2804, 2.9181) (113.7405, 1.6531) (118.1824, 0.3262) knots 0 0 0 0 1 1 1 1
  spline S255 degree 3 poles (132.6089, 28.3194) (132.2808, 27.9912) (131.8358, 27.8068) (131.3718, 27.8067) knots 0 0 0 0 1 1 1 1
  spline S256 degree 3 poles (129.6215, 29.557) (129.6216, 30.021) (129.806, 30.466) (130.1341, 30.7941) knots 0 0 0 0 1 1 1 1
  line L93 (105.4933, 31.1574) -> (106.8022, 31.1114)
  spline S257 degree 3 poles (110.8438, 38.2748) (110.729, 38.1158) (110.6529, 37.9321) (110.6216, 37.7384) knots 0 0 0 0 1 1 1 1
  spline S258 degree 3 poles (110.9906, 36.8475) (111.2268, 36.6111) (111.5473, 36.4782) (111.8815, 36.478) knots 0 0 0 0 1 1 1 1
  spline S259 degree 3 poles (112.7724, 36.8475) (113.0089, 37.0837) (113.1418, 37.4042) (113.1419, 37.7384) knots 0 0 0 0 1 1 1 1
  spline S260 degree 3 poles (107.4151, 39.714) (107.2591, 39.8042) (107.092, 39.8735) (106.918, 39.9202) knots 0 0 0 0 1 1 1 1
  spline S261 degree 3 poles (50.3876, 15.5393) (54.9707, 14.841) (59.5438, 14.0791) (64.1056, 13.2536) knots 0 0 0 0 1 1 1 1
  spline S262 degree 3 poles (107.4151, 36.1463) (107.5711, 36.2362) (107.7146, 36.3462) (107.842, 36.4734) knots 0 0 0 0 1 1 1 1
  spline S263 degree 3 poles (119.5777, 0.0839) (120.0506, 0.0585) (120.5248, 0.0892) (120.9905, 0.1753) knots 0 0 0 0 1 1 1 1
  spline S264 degree 3 poles (106.3852, 39.9905) (105.8388, 39.9905) (105.3148, 39.7733) (104.9284, 39.3869) knots 0 0 0 0 1 1 1 1
  spline S265 degree 3 poles (125.3241, 3.2609) (125.5725, 3.5801) (125.8182, 3.9013) (126.061, 4.2247) knots 0 0 0 0 1 1 1 1
  spline S266 degree 3 poles (130.1341, 30.7941) (130.4624, 31.1224) (130.9076, 31.3068) (131.3718, 31.3068) knots 0 0 0 0 1 1 1 1
  spline S267 degree 3 poles (118.1824, 0.3262) (118.6363, 0.1907) (119.1047, 0.1093) (119.5777, 0.0839) knots 0 0 0 0 1 1 1 1
  spline S268 degree 3 poles (104.9284, 39.3869) (104.542, 39.0006) (104.3249, 38.4766) (104.3249, 37.9301) knots 0 0 0 0 1 1 1 1
  spline S269 degree 3 poles (106.8022, 31.1114) (107.1237, 31.1002) (107.4267, 31.2614) (107.597, 31.5342) knots 0 0 0 0 1 1 1 1
  spline S270 degree 3 poles (104.9284, 36.4734) (105.3148, 36.0871) (105.8389, 35.8702) (106.3852, 35.8703) knots 0 0 0 0 1 1 1 1
  spline S271 degree 3 poles (104.7626, 32.5331) (104.5926, 32.2605) (104.5808, 31.918) (104.7316, 31.6344) knots 0 0 0 0 1 1 1 1
  spline S272 degree 3 poles (107.597, 31.5342) (107.7673, 31.8067) (107.7793, 32.1495) (107.6285, 32.4333) knots 0 0 0 0 1 1 1 1
  spline S273 degree 3 poles (105.5558, 32.9563) (105.2348, 32.9668) (104.9325, 32.8056) (104.7626, 32.5331) knots 0 0 0 0 1 1 1 1
  spline S274 degree 3 poles (137.3523, 26.9101) (137.464, 27.2988) (137.5724, 27.6885) (137.6773, 28.0791) knots 0 0 0 0 1 1 1 1
  spline S275 degree 3 poles (137.6773, 28.0791) (137.7822, 28.4697) (137.8837, 28.8613) (137.9817, 29.2537) knots 0 0 0 0 1 1 1 1
  spline S276 degree 3 poles (139.379, 36.3954) (139.4359, 36.7957) (139.4893, 37.1966) (139.5392, 37.5979) knots 0 0 0 0 1 1 1 1
  spline S277 degree 3 poles (135.8511, 22.2954) (135.9894, 22.6756) (136.1245, 23.057) (136.2562, 23.4396) knots 0 0 0 0 1 1 1 1
  spline S278 degree 3 poles (139.5392, 37.5979) (139.5891, 37.9992) (139.6354, 38.4009) (139.6783, 38.803) knots 0 0 0 0 1 1 1 1
  spline S279 degree 3 poles (139.6783, 38.803) (139.7214, 39.2052) (139.761, 39.6077) (139.7971, 40.0106) knots 0 0 0 0 1 1 1 1
  spline S280 degree 3 poles (137.0071, 25.7469) (137.1255, 26.1336) (137.2406, 26.5214) (137.3523, 26.9101) knots 0 0 0 0 1 1 1 1
  spline S281 degree 3 poles (138.2659, 30.4329) (138.3574, 30.827) (138.4454, 31.2218) (138.53, 31.6173) knots 0 0 0 0 1 1 1 1
  spline S282 degree 3 poles (139.9713, 42.4312) (139.9932, 42.8349) (140.0116, 43.2389) (140.0266, 43.643) knots 0 0 0 0 1 1 1 1
  spline S283 degree 3 poles (138.53, 31.6173) (138.6146, 32.013) (138.6957, 32.4094) (138.7734, 32.8064) knots 0 0 0 0 1 1 1 1
  spline S284 degree 3 poles (135.4263, 21.1591) (135.5712, 21.5366) (135.7128, 21.9154) (135.8511, 22.2954) knots 0 0 0 0 1 1 1 1
  spline S285 degree 3 poles (134.5173, 18.9091) (134.6753, 19.2815) (134.8299, 19.6553) (134.9814, 20.0305) knots 0 0 0 0 1 1 1 1
  spline S286 degree 3 poles (136.2562, 23.4396) (136.3881, 23.8219) (136.5166, 24.2053) (136.6417, 24.5899) knots 0 0 0 0 1 1 1 1
  spline S287 degree 3 poles (134.9814, 20.0305) (135.133, 20.4054) (135.2813, 20.7816) (135.4263, 21.1591) knots 0 0 0 0 1 1 1 1
  spline S288 degree 3 poles (136.6417, 24.5899) (136.7669, 24.9745) (136.8887, 25.3602) (137.0071, 25.7469) knots 0 0 0 0 1 1 1 1
  spline S289 degree 3 poles (137.9817, 29.2537) (138.0799, 29.6459) (138.1746, 30.039) (138.2659, 30.4329) knots 0 0 0 0 1 1 1 1
  spline S290 degree 3 poles (138.7734, 32.8064) (138.8509, 33.2033) (138.925, 33.6009) (138.9956, 33.9991) knots 0 0 0 0 1 1 1 1
  spline S291 degree 3 poles (138.9956, 33.9991) (139.0664, 34.3973) (139.1338, 34.7961) (139.1977, 35.1954) knots 0 0 0 0 1 1 1 1
  spline S292 degree 3 poles (139.1977, 35.1954) (139.2616, 35.5949) (139.3221, 35.9949) (139.379, 36.3954) knots 0 0 0 0 1 1 1 1
  spline S293 degree 3 poles (139.7971, 40.0106) (139.8332, 40.4134) (139.8657, 40.8165) (139.8948, 41.2199) knots 0 0 0 0 1 1 1 1
  spline S294 degree 3 poles (139.8948, 41.2199) (139.9238, 41.6234) (139.9493, 42.0272) (139.9713, 42.4312) knots 0 0 0 0 1 1 1 1
  spline S295 degree 3 poles (140.0674, 47.2825) (140.0614, 47.6869) (140.0519, 48.0912) (140.039, 48.4954) knots 0 0 0 0 1 1 1 1
  spline S296 degree 3 poles (44.6267, 89.6179) (41.8809, 89.2657) (39.1426, 88.8565) (36.4138, 88.3906) knots 0 0 0 0 1 1 1 1
  spline S297 degree 3 poles (140.0266, 43.643) (140.0416, 44.0471) (140.0531, 44.4514) (140.0612, 44.8558) knots 0 0 0 0 1 1 1 1
  spline S298 degree 3 poles (135.97, 69.8636) (135.8334, 70.2443) (135.6935, 70.6238) (135.5503, 71.002) knots 0 0 0 0 1 1 1 1
  spline S299 degree 3 poles (133.1613, 76.5763) (132.9862, 76.941) (132.8079, 77.3041) (132.6265, 77.6657) knots 0 0 0 0 1 1 1 1
  spline S300 degree 3 poles (132.6265, 77.6657) (132.445, 78.0271) (132.2603, 78.387) (132.0725, 78.7452) knots 0 0 0 0 1 1 1 1
  spline S301 degree 3 poles (140.039, 48.4954) (140.0259, 48.8996) (140.0094, 49.3038) (139.9893, 49.7077) knots 0 0 0 0 1 1 1 1
  spline S302 degree 3 poles (69.4722, 91.2426) (66.7039, 91.2343) (63.936, 91.1685) (61.1704, 91.0452) knots 0 0 0 0 1 1 1 1
  spline S303 degree 3 poles (133.6781, 75.4787) (133.509, 75.8461) (133.3368, 76.212) (133.1613, 76.5763) knots 0 0 0 0 1 1 1 1
  spline S304 degree 3 poles (140.0746, 46.0692) (140.0757, 46.4736) (140.0733, 46.8781) (140.0674, 47.2825) knots 0 0 0 0 1 1 1 1
  spline S305 degree 3 poles (28.2587, 86.8233) (25.5514, 86.2443) (22.8564, 85.6093) (20.1755, 84.9185) knots 0 0 0 0 1 1 1 1
  spline S306 degree 3 poles (20.1755, 84.9185) (17.4947, 84.2279) (14.8284, 83.4817) (12.1786, 82.6804) knots 0 0 0 0 1 1 1 1
  spline S307 degree 3 poles (140.0612, 44.8558) (140.0692, 45.2602) (140.0736, 45.6647) (140.0746, 46.0692) knots 0 0 0 0 1 1 1 1
  spline S308 degree 3 poles (138.6018, 60.5282) (138.5193, 60.9243) (138.4333, 61.3196) (138.344, 61.7142) knots 0 0 0 0 1 1 1 1
  spline S309 degree 3 poles (134.1752, 74.3718) (134.0127, 74.7422) (133.847, 75.1112) (133.6781, 75.4787) knots 0 0 0 0 1 1 1 1
  spline S310 degree 3 poles (139.9185, 50.919) (139.8916, 51.3225) (139.8611, 51.7258) (139.8271, 52.1288) knots 0 0 0 0 1 1 1 1
  spline S311 degree 3 poles (9.5627, 81.067) (9.2059, 80.6908) (8.8993, 80.2699) (8.6506, 79.8149) knots 0 0 0 0 1 1 1 1
  spline S312 degree 3 poles (12.1786, 82.6804) (11.6821, 82.5301) (11.2072, 82.3161) (10.7657, 82.0437) knots 0 0 0 0 1 1 1 1
  spline S313 degree 3 poles (10.7657, 82.0437) (10.3242, 81.7715) (9.9198, 81.4432) (9.5627, 81.067) knots 0 0 0 0 1 1 1 1
  spline S314 degree 3 poles (8.6506, 79.8149) (7.8156, 78.2871) (7.0378, 76.7287) (6.319, 75.1428) knots 0 0 0 0 1 1 1 1
  spline S315 degree 3 poles (139.8271, 52.1288) (139.7932, 52.5318) (139.7558, 52.9345) (139.7149, 53.3369) knots 0 0 0 0 1 1 1 1
  spline S316 degree 3 poles (123.303, 84.0689) (121.8117, 84.4807) (120.3125, 84.8632) (118.8061, 85.2161) knots 0 0 0 0 1 1 1 1
  spline S317 degree 3 poles (132.0725, 78.7452) (131.8846, 79.1034) (131.6935, 79.46) (131.4994, 79.8149) knots 0 0 0 0 1 1 1 1
  spline S318 degree 3 poles (139.2519, 56.9471) (139.1901, 57.3467) (139.1248, 57.7459) (139.0561, 58.1444) knots 0 0 0 0 1 1 1 1
  spline S319 degree 3 poles (6.319, 75.1428) (5.6003, 73.5572) (4.9409, 71.9454) (4.3424, 70.3106) knots 0 0 0 0 1 1 1 1
  spline S320 degree 3 poles (1.495, 60.2714) (1.1461, 58.5658) (0.861, 56.8477) (0.6403, 55.1208) knots 0 0 0 0 1 1 1 1
  spline S321 degree 3 poles (134.6527, 73.2567) (134.4968, 73.6298) (134.3376, 74.0015) (134.1752, 74.3718) knots 0 0 0 0 1 1 1 1
  spline S322 degree 3 poles (127.9715, 82.6804) (127.8983, 82.7025) (127.8251, 82.7245) (127.7519, 82.7465) knots 0 0 0 0 1 1 1 1
  spline S323 degree 3 poles (110.7121, 87.0718) (108.0014, 87.6344) (105.2794, 88.1406) (102.5477, 88.5901) knots 0 0 0 0 1 1 1 1
  spline S324 degree 3 poles (139.9893, 49.7077) (139.9692, 50.1117) (139.9456, 50.5155) (139.9185, 50.919) knots 0 0 0 0 1 1 1 1
  spline S325 degree 3 poles (137.7667, 64.0712) (137.6638, 64.4622) (137.5576, 64.8524) (137.4479, 65.2416) knots 0 0 0 0 1 1 1 1
  spline S326 degree 3 poles (138.8395, 59.3386) (138.7637, 59.7359) (138.6845, 60.1324) (138.6018, 60.5282) knots 0 0 0 0 1 1 1 1
  spline S327 degree 3 poles (2.7316, 65.344) (2.2565, 63.6691) (1.844, 61.977) (1.495, 60.2714) knots 0 0 0 0 1 1 1 1
  spline S328 degree 3 poles (136.3694, 68.7179) (136.2396, 69.101) (136.1064, 69.4829) (135.97, 69.8636) knots 0 0 0 0 1 1 1 1
  spline S329 degree 3 poles (139.7149, 53.3369) (139.6738, 53.7394) (139.6292, 54.1414) (139.5811, 54.5431) knots 0 0 0 0 1 1 1 1
  spline S330 degree 3 poles (138.0659, 62.895) (137.9696, 63.2879) (137.8699, 63.68) (137.7667, 64.0712) knots 0 0 0 0 1 1 1 1
  spline S331 degree 3 poles (130.5873, 81.067) (130.2302, 81.4432) (129.8259, 81.7715) (129.3843, 82.0437) knots 0 0 0 0 1 1 1 1
  spline S332 degree 3 poles (4.3424, 70.3106) (3.7439, 68.6757) (3.2066, 67.019) (2.7316, 65.344) knots 0 0 0 0 1 1 1 1
  spline S333 degree 3 poles (0.6403, 55.1208) (0.4194, 53.3938) (0.2631, 51.6592) (0.1716, 49.9206) knots 0 0 0 0 1 1 1 1
  spline S334 degree 3 poles (137.1084, 66.4064) (136.9918, 66.7938) (136.872, 67.1802) (136.7487, 67.5655) knots 0 0 0 0 1 1 1 1
  spline S335 degree 3 poles (135.5503, 71.002) (135.4074, 71.3803) (135.2611, 71.7574) (135.1116, 72.1332) knots 0 0 0 0 1 1 1 1
  spline S336 degree 3 poles (0.1716, 49.9206) (0.0801, 48.1821) (0.0536, 46.4408) (0.092, 44.7003) knots 0 0 0 0 1 1 1 1
  spline S337 degree 3 poles (138.344, 61.7142) (138.2547, 62.1086) (138.162, 62.5022) (138.0659, 62.895) knots 0 0 0 0 1 1 1 1
  spline S338 degree 3 poles (52.8836, 90.5031) (50.1255, 90.2652) (47.3726, 89.9701) (44.6267, 89.6179) knots 0 0 0 0 1 1 1 1
  spline S339 degree 3 poles (139.0561, 58.1444) (138.9873, 58.5431) (138.9152, 58.9412) (138.8395, 59.3386) knots 0 0 0 0 1 1 1 1
  spline S340 degree 3 poles (61.1704, 91.0452) (58.4047, 90.9219) (55.6418, 90.7412) (52.8836, 90.5031) knots 0 0 0 0 1 1 1 1
  spline S341 degree 3 poles (136.7487, 67.5655) (136.6256, 67.9507) (136.4992, 68.3349) (136.3694, 68.7179) knots 0 0 0 0 1 1 1 1
  spline S342 degree 3 poles (135.1116, 72.1332) (134.9619, 72.509) (134.8089, 72.8835) (134.6527, 73.2567) knots 0 0 0 0 1 1 1 1
  spline S343 degree 3 poles (137.4479, 65.2416) (137.3381, 65.6309) (137.2249, 66.0192) (137.1084, 66.4064) knots 0 0 0 0 1 1 1 1
  spline S344 degree 3 poles (139.5811, 54.5431) (139.5332, 54.9447) (139.4819, 55.3459) (139.4271, 55.7466) knots 0 0 0 0 1 1 1 1
  spline S345 degree 3 poles (127.7519, 82.7465) (126.2777, 83.2164) (124.7945, 83.6573) (123.303, 84.0689) knots 0 0 0 0 1 1 1 1
  spline S346 degree 3 poles (131.4994, 79.8149) (131.2508, 80.2699) (130.9442, 80.6908) (130.5873, 81.067) knots 0 0 0 0 1 1 1 1
  spline S347 degree 3 poles (129.3843, 82.0437) (128.9429, 82.3161) (128.468, 82.5301) (127.9715, 82.6804) knots 0 0 0 0 1 1 1 1
  spline S348 degree 3 poles (118.8061, 85.2161) (116.1213, 85.8906) (113.4226, 86.5093) (110.7121, 87.0718) knots 0 0 0 0 1 1 1 1
  spline S349 degree 3 poles (36.4138, 88.3906) (33.6849, 87.9247) (30.9659, 87.4021) (28.2587, 86.8233) knots 0 0 0 0 1 1 1 1